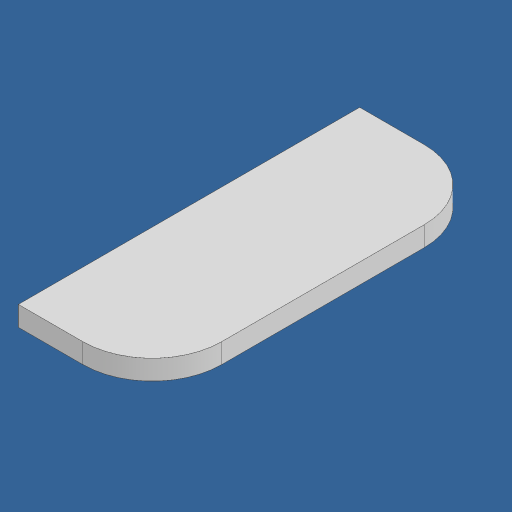
# Autodesk Inventor part: Fan_Duct_2A
Saved by Autodesk Inventor 2024.2 (Build 282272000, 272)
## iProperties
Created: 2024-06-09
Part Number: Fan_Duct_2A
Material: Generic
Document SubType Name: Modeling
Designer: Charlie Kendall
Density: 1 g/cm^3
Appearance: Default
Author: Charlie Kendall
Autodesk Inventor part; units mm, degrees
ref_plane "YZ Plane" through (0, 0, 0) normal (1, 0, 0) x (0, 1, 0)
ref_plane "XZ Plane" through (0, 0, 0) normal (0, 1, 0) x (-1, 0, 0)
ref_plane "XY Plane" through (0, 0, 0) normal (0, 0, 1) x (1, 0, 0)
sketch "Sketch1" plane through (0, 0, 0) normal (0, 1, 0) x (-1, 0, 0)
  line L0 (6.75, 17.2) -> (-6.75, 17.2)
  line L1 (-6.75, 17.2) -> (-6.75, -17.2)
  line L2 (-6.75, -17.2) -> (6.75, -17.2)
  line L3 (6.75, -17.2) -> (6.75, 17.2)
  line L4 (6.75, 17.2) -> (-6.75, -17.2) construction
  line L5 (-6.75, 17.2) -> (6.75, -17.2) construction
  point P0 (0, 0)
  dimension "d0" = 34.4
  dimension "d1" = 13.5
  constraints: 12 end point, 2 midpoint, 2 parallel, 1 horizontal, 1 perpendicular
  measures "d0" distance of L2.end L0.start
  measures "d1" distance of L1.end L2.end
extrude "Extrusion1" add sketch "Sketch1" against normal blind 2
fillet "Fillet1" radius 7 2 edges at (6.75, -1, 17.2) (6.75, -1, -17.2)
body "Solid1"
